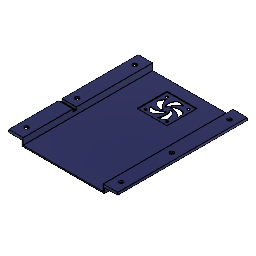
1-CBA bottom Cover V3 - part 2of3 v1 v5 (Autodesk Fusion 360 design; units mm, degrees)
Autodesk Fusion 360 part; units mm, degrees
note: some values were not read from the file. Set by a fixed rule: which sketch regions a step uses.
sketch "extrusion" plane through (0, 0, 0) normal (0, 1, 0) x (1, 0, 0)
  line L0 (-82.5, -8) -> (-62.5, -8)
  line L1 (-62.5, -8) -> (-62.5, 0)
  line L2 (-62.5, 0) -> (62.5, 0)
  line L3 (62.5, 0) -> (62.5, -8)
  line L4 (62.5, -8) -> (82.5, -8)
  line L5 (-60.5, -12) -> (-60.5, -2)
  line L6 (-60.5, -2) -> (60.5, -2)
  line L7 (60.5, -2) -> (60.5, -12)
  line L8 (-82.5, -12) -> (-60.5, -12)
  line L9 (60.5, -12) -> (82.5, -12)
  line L10 (-82.5, -8) -> (-82.5, -12)
  line L11 (82.5, -8) -> (82.5, -12)
  dimension "d1" = 125
  dimension "d2" = 8
  dimension "d3" = 20
  dimension "d4" = 8
  dimension "d5" = 20
  constraint horizontal L0
  constraint perpendicular L0 L1
  constraint perpendicular L1 L2
  constraint perpendicular L2 L3
  constraint perpendicular L1 L4
  constraint midpoint origin L2
  constraint parallel L1 L5
  constraint parallel L2 L6
  constraint parallel L3 L7
  constraint parallel L4 L9
  constraint parallel L0 L8
  constraint perpendicular L8 L10
  constraint perpendicular L9 L11
  measures "d1" distance of L1.end L2.end
  measures "d2" distance of L0.end L1.end
  measures "d3" distance of L0.start L0.end
  measures "d4" distance of L2.end L3.end
  measures "d5" distance of L3.end L4.end
extrude "Extrude1" add sketch "extrusion" along normal mid plane 196
sketch "top holes" plane through (0, 0, 12) normal (0, 0, 1) x (-1, 0, 0)
  circle A0 centre (71.5, -81.75) radius 3
  line L0 (82.5, -98) -> (60.5, -98)
  point P0 (71.5, -98)
  dimension "d11" = 6
  dimension "d12" = 16.25
  constraint midpoint L0 P0
  constraint vertical A0.centre P0
  measures "d11" diameter of A0
  measures "d12" distance of A0.centre L0
extrude "Extrude2" cut sketch "top holes" against normal blind 4
mirror "Mirror1" about plane through (0, 0, 0) normal (1, 0, 0) of "Extrude2"
mirror "Mirror2" about plane through (0, 0, 0) normal (0, 1, 0) of "Extrude2", "Mirror1"
sketch "square undent" plane through (0, 0, 2) normal (0, 0, 1) x (-1, 0, 0)
  line L0 (22.5, -81.5) -> (-22.5, -81.5)
  line L1 (-22.5, -81.5) -> (-22.5, -36.5)
  line L2 (-22.5, -36.5) -> (22.5, -36.5)
  line L3 (22.5, -36.5) -> (22.5, -81.5)
  line L4 (60.5, -98) -> (-60.5, -98)
  point P0 (0, -81.5)
  dimension "d17" = 45
  dimension "d18" = 45
  dimension "d19" = 16.5
  constraint horizontal L0
  constraint vertical L1
  constraint horizontal L2
  constraint vertical L3
  constraint midpoint L0 P0
  constraint vertical origin P0
  measures "d17" distance of L0.start L0.end
  measures "d18" distance of L0.start L2.end
  measures "d19" distance of L0.start L4
extrude "Extrude3" cut sketch "square undent" against normal blind 1
sketch "square holes" plane through (0, 0, 1) normal (0, 0, 1) x (-1, 0, 0)
  circle A0 centre (16.1, -75.1) radius 1.75
  line L0 (22.5, -81.5) -> (-22.5, -81.5)
  line L1 (22.5, -36.5) -> (22.5, -81.5)
  line L2 (-22.5, -36.5) -> (22.5, -81.5) construction
  circle A1 centre (0, -59) radius 18.5
  arc A2 (-16.7163, -66.9255) -> (-0.2693, -65.0246) centre (-10.0258, -52.7122) ccw
  arc A3 (-0.2693, -65.0246) -> (-1.0892, -63.2504) centre (-0.8821, -64.2312) ccw
  arc A4 (-18.3833, -56.9255) -> (-1.0892, -63.2504) centre (-3.6534, -43.4554) ccw
  point P0 (-22.5, -36.5)
  dimension "d22" = 3.5
  dimension "d23" = 6.4
  dimension "d24" = 6.4
  dimension "d25" = 37
  dimension "d66" = 10
  constraint coincident P0 L2.start
  constraint coincident L0.start L1.end
  constraint midpoint L2 A1.centre
  constraint coincident A1 A2.start
  constraint coincident A1 A4.start
  measures "d22" diameter of A0
  measures "d23" distance of A0.centre L0
  measures "d24" distance of A0.centre L1
  measures "d25" diameter of A1
  measures "d66" vertical distance of A2.start A4.start
extrude "Extrude4" cut sketch "square holes" against normal blind 1 contours A0
ref_plane "WorkPlane1" through (0, 59, 1.5) normal (0, -1, 0) x (-1, 0, 0)
mirror "Mirror3" about plane through (0, 59, 1.5) normal (0, -1, 0) of "Extrude4"
mirror "Mirror4" about plane through (0, 0, 0) normal (1, 0, 0) of "Extrude4", "Mirror3"
extrude "Extrude5" cut sketch "square holes" against normal blind 1 contours A1 A2 A3 A4 picked at (-14.7047, -64.6465)
pattern_circular "C-Pattern1" count 5 over 360 about axis through (0, 59, 1) along (0, 0, -1) of "Extrude5"
sketch "midhole" plane through (0, 0, 12) normal (0, 0, 1) x (-1, 0, 0)
  circle A0 centre (71.5, 5.25) radius 3
  circle A1 centre (71.5, -81.75) radius 3
  dimension "d40" = 81
  constraint equal A0 A1
  constraint vertical A0.centre A1.centre
  measures "d40" distance of A0 A1
extrude "Extrude6" cut sketch "midhole" against normal blind 4 contours A0
mirror "Mirror5" about plane through (0, 0, 0) normal (1, 0, 0) of "Extrude6"
sketch "Sketch6" plane through (0, 0, 12) normal (0, 0, 1) x (-1, 0, 0)
  line L0 (60.5, 22.5) -> (82.5, 22.5)
  line L1 (82.5, 22.5) -> (82.5, 17.5)
  line L2 (82.5, 17.5) -> (60.5, 17.5)
  line L3 (60.5, 17.5) -> (60.5, 22.5)
  line L4 (60.5, 98) -> (60.5, -98)
  line L5 (82.5, 98) -> (82.5, -98)
  line L6 (60.5, 98) -> (82.5, 98)
  dimension "d44" = 5
  dimension "d45" = 75.5
  constraint horizontal L0
  constraint vertical L1
  constraint horizontal L2
  constraint vertical L3
  constraint coincident L1.end L5
  constraint coincident L0.start L4
  measures "d44" distance of L0.start L2.end
  measures "d45" distance of L0 L6
extrude "Extrude7" cut sketch "Sketch6" against normal blind 4 contours L0 L1 L2 L3 L4 L5
sketch "Sketch7" plane through (0, 0, 8) normal (0, 0, -1) x (1, 0, 0)
  line L0 (-82.5, 22.5) -> (-62.5, 22.5)
  line L1 (-62.5, 22.5) -> (-62.5, 98)
  line L2 (-62.5, 98) -> (-82.5, 98)
  line L3 (-82.5, 98) -> (-82.5, 22.5)
  circle A0 centre (-71.5, 81.75) radius 3
  circle A1 centre (-71.5, 81.75) radius 5
  dimension "d48" = 10
  constraint concentric A0 A1
  measures "d48" diameter of A1
extrude "Extrude8" cut sketch "Sketch7" against normal blind 2 contours A1
sketch "Sketch8" plane through (0, 0, 8) normal (0, 0, -1) x (1, 0, 0)
  line L0 (-62.5, 17.5) -> (-82.5, 17.5)
  line L1 (-82.5, 17.5) -> (-82.5, -98)
  line L2 (-82.5, -98) -> (-62.5, -98)
  line L3 (-62.5, -98) -> (-62.5, 17.5)
  circle A0 centre (-71.5, -81.75) radius 3
  circle A1 centre (-71.5, 5.25) radius 3
  circle A2 centre (-71.5, 5.25) radius 5
  dimension "d51" = 10
  constraint concentric A1 A2
  measures "d51" diameter of A2
extrude "Extrude9" cut sketch "Sketch8" against normal blind 2 contours A2
sketch "Sketch9" plane through (0, 0, 8) normal (0, 0, -1) x (1, 0, 0)
  circle A0 centre (-71.5, 5.25) radius 5
  line L0 (-62.5, 17.5) -> (-82.5, 17.5)
  line L1 (-82.5, 17.5) -> (-82.5, -98)
  line L2 (-82.5, -98) -> (-62.5, -98)
  line L3 (-62.5, -98) -> (-62.5, 17.5)
  circle A1 centre (-71.5, -81.75) radius 3
  circle A2 centre (-71.5, -81.75) radius 5
  dimension "d54" = 10
  constraint concentric A1 A2
  measures "d54" diameter of A2
extrude "Extrude10" cut sketch "Sketch9" against normal blind 2 contours A2
sketch "Sketch10" plane through (0, 0, 8) normal (0, 0, -1) x (1, 0, 0)
  circle A0 centre (71.5, 5.25) radius 3
  circle A1 centre (71.5, 81.75) radius 3
  circle A2 centre (71.5, -81.75) radius 3
  line L0 (62.5, 98) -> (62.5, -98)
  line L1 (62.5, -98) -> (82.5, -98)
  line L2 (82.5, -98) -> (82.5, 98)
  line L3 (82.5, 98) -> (62.5, 98)
  circle A3 centre (71.5, 81.75) radius 5
  dimension "d57" = 10
  constraint concentric A1 A3
  measures "d57" diameter of A3
extrude "Extrude11" cut sketch "Sketch10" against normal blind 2 contours A3
sketch "Sketch11" plane through (0, 0, 8) normal (0, 0, -1) x (1, 0, 0)
  circle A0 centre (71.5, 81.75) radius 5
  circle A1 centre (71.5, 5.25) radius 3
  circle A2 centre (71.5, -81.75) radius 3
  line L0 (62.5, 98) -> (62.5, -98)
  line L1 (62.5, -98) -> (82.5, -98)
  line L2 (82.5, -98) -> (82.5, 98)
  line L3 (82.5, 98) -> (62.5, 98)
  circle A3 centre (71.5, 5.25) radius 5
  dimension "d60" = 10
  constraint concentric A1 A3
  measures "d60" diameter of A3
extrude "Extrude12" cut sketch "Sketch11" against normal blind 2 contours A3
sketch "Sketch12" plane through (0, 0, 8) normal (0, 0, -1) x (1, 0, 0)
  circle A0 centre (71.5, 5.25) radius 5
  circle A1 centre (71.5, 81.75) radius 5
  circle A2 centre (71.5, -81.75) radius 3
  line L0 (62.5, 98) -> (62.5, -98)
  line L1 (62.5, -98) -> (82.5, -98)
  line L2 (82.5, -98) -> (82.5, 98)
  line L3 (82.5, 98) -> (62.5, 98)
  circle A3 centre (71.5, -81.75) radius 5
  dimension "d63" = 10
  constraint concentric A2 A3
  measures "d63" diameter of A3
extrude "Extrude13" cut sketch "Sketch12" against normal blind 2 contours A3
